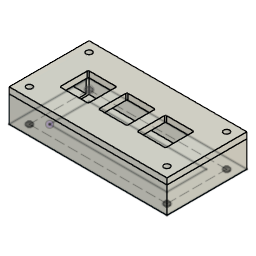
PCBT1 (Autodesk Fusion 360 design; units mm, degrees)
part number: 2026-06-29-22-35-08-349
Autodesk Fusion 360 part; units mm, degrees
sketch "Sketch1" plane through (0, 0, 0) normal (0, 0, 1) x (1, 0, 0)
  line L0 (0, 0) -> (57.8, 0)
  line L1 (57.8, 0) -> (57.8, 19.4)
  line L2 (57.8, 19.4) -> (0, 19.4)
  line L3 (0, 19.4) -> (0, 0)
  line L4 (-10, -10) -> (67.8, -10)
  line L5 (67.8, -10) -> (67.8, 29.4)
  line L6 (67.8, 29.4) -> (-10, 29.4)
  line L7 (-10, 29.4) -> (-10, -10)
  line L8 (-5, -5) -> (62.8, -5) construction
  line L9 (62.8, -5) -> (62.8, 24.4) construction
  line L10 (62.8, 24.4) -> (-5, 24.4) construction
  line L11 (-5, 24.4) -> (-5, -5) construction
  circle A0 centre (-5, 24.4) radius 1.45
  circle A1 centre (62.8, 24.4) radius 1.45
  circle A2 centre (62.8, -5) radius 1.45
  circle A3 centre (-5, -5) radius 1.45
  point P0 (-5, 24.4)
  dimension "d1" = 57.8
  dimension "d2" = 19.4
  dimension "d7" = 10
  dimension "d8" = 5
  dimension "d9" = 2.9
  dimension "d10" = 2.9
  dimension "d11" = 2.9
  dimension "d12" = 2.9
  constraint horizontal L0
  constraint vertical L1
  constraint horizontal L2
  constraint vertical L3
  constraint coincident L0.start L3.end
  constraint coincident P0 L10.end
  constraint coincident L9.end L10.start
  constraint coincident L8.end L9.start
  constraint coincident L8.start L11.end
  measures "d1" distance of L0.start L0.end
  measures "d2" distance of L0.start L2.end
  measures "d9" diameter of A0
  measures "d10" diameter of A1
  measures "d11" diameter of A2
  measures "d12" diameter of A3
extrude "Extrude1" add sketch "Sketch1" along normal blind 3 contours L0 L1 L2 L3 makes body 1
extrude "Extrude2" add sketch "Sketch1" along normal blind 13 bodies 1
sketch "plate-2026-06-29T21_50_33.352Z" plane through (0, 0, 13) normal (0, 0, 1) x (1, 0, 0)
  line L0 (3.025, 16.475) -> (16.025, 16.475)
  line L1 (3.025, 2.475) -> (16.025, 2.475)
  line L2 (2.525, 15.975) -> (2.525, 2.975)
  line L3 (16.525, 15.975) -> (16.525, 2.975)
  arc A0 (3.025, 16.475) -> (2.525, 15.975) centre (3.025, 15.975) ccw
  arc A1 (16.525, 15.975) -> (16.025, 16.475) centre (16.025, 15.975) ccw
  arc A2 (2.525, 2.975) -> (3.025, 2.475) centre (3.025, 2.975) ccw
  arc A3 (16.025, 2.475) -> (16.525, 2.975) centre (16.025, 2.975) ccw
  line L4 (22.075, 16.475) -> (35.075, 16.475)
  line L5 (22.075, 2.475) -> (35.075, 2.475)
  line L6 (21.575, 15.975) -> (21.575, 2.975)
  line L7 (35.575, 15.975) -> (35.575, 2.975)
  arc A4 (22.075, 16.475) -> (21.575, 15.975) centre (22.075, 15.975) ccw
  arc A5 (35.575, 15.975) -> (35.075, 16.475) centre (35.075, 15.975) ccw
  arc A6 (21.575, 2.975) -> (22.075, 2.475) centre (22.075, 2.975) ccw
  arc A7 (35.075, 2.475) -> (35.575, 2.975) centre (35.075, 2.975) ccw
  line L8 (41.125, 16.475) -> (54.125, 16.475)
  line L9 (41.125, 2.475) -> (54.125, 2.475)
  line L10 (40.625, 15.975) -> (40.625, 2.975)
  line L11 (54.625, 15.975) -> (54.625, 2.975)
  arc A8 (41.125, 16.475) -> (40.625, 15.975) centre (41.125, 15.975) ccw
  arc A9 (54.625, 15.975) -> (54.125, 16.475) centre (54.125, 15.975) ccw
  arc A10 (40.625, 2.975) -> (41.125, 2.475) centre (41.125, 2.975) ccw
  arc A11 (54.125, 2.475) -> (54.625, 2.975) centre (54.125, 2.975) ccw
  line L12 (0, -0.05) -> (58, 0)
  line L13 (0, 20) -> (58, 20)
  line L14 (0, -0.05) -> (0, 20)
  line L15 (58, 0) -> (58, 20)
extrude "Extrude3" add sketch "plate-2026-06-29T21_50_33.352Z" 1 faces at (19.2667, -3.7528, 13) along normal blind 3 separate body on bodies 1 makes body 2
sketch "Sketch3" plane through (-10, 0, 0) normal (-1, 0, 0) x (0, -1, 0)
  line L0 (-29.4, 0) -> (10, 0)
  line L1 (10, 0) -> (10, 13)
  line L2 (10, 13) -> (-29.4, 13)
  line L3 (-29.4, 13) -> (-29.4, 0)
sketch "Sketch4" plane through (-10, 0, 0) normal (-1, 0, 0) x (0, -1, 0)
  line L0 (-18, 13) -> (-2, 13) construction
  line L1 (-2, 13) -> (-2, 4) construction
  line L2 (-2, 4) -> (-18, 4) construction
  line L3 (-18, 4) -> (-18, 13) construction
  line L4 (-18, 13) -> (-2, 13)
  line L5 (-2, 13) -> (-2, 4)
  line L6 (-2, 4) -> (-18, 4)
  line L7 (-18, 4) -> (-18, 13)
  constraint horizontal L0
  constraint vertical L1
  constraint horizontal L2
  constraint vertical L3
  constraint horizontal L4
  constraint vertical L5
  constraint horizontal L6
  constraint vertical L7
extrude "Extrude4" cut sketch "Sketch4" against normal blind 10 bodies 1
